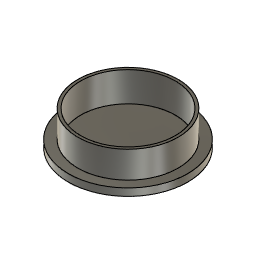
PVC End Cap v1 (Autodesk Fusion 360 design; units mm, degrees)
Autodesk Fusion 360 part; units mm, degrees
sketch "Sketch1" plane through (0, 0, 0) normal (0, 0, 1) x (1, 0, 0)
  circle A0 centre (0, 0) radius 30.235
  dimension "d1" = 60.47
  constraint coincident A0.centre origin
  measures "d1" diameter of A0
extrude "Extrude1" add sketch "Sketch1" along normal blind 3.72
sketch "Sketch2" plane through (0, 0, 3.72) normal (0, 0, 1) x (-1, 0, 0)
  circle A0 centre (0, 0) radius 30.235
  circle A1 centre (0, 0) radius 25.4
  dimension "d4" = 50.8
  constraint coincident A0.centre A1.centre
  measures "d4" diameter of A1
extrude "Extrude2" add sketch "Sketch2" along normal blind 13.57 contours A1
sketch "Sketch3" plane through (0, 0, 17.29) normal (0, 0, 1) x (-1, 0, 0)
  circle A0 centre (0, 0) radius 25.4
  circle A1 centre (0, 0) radius 24
  dimension "d10" = 48
  constraint coincident A0.centre A1.centre
  measures "d10" diameter of A1
extrude "Extrude3" cut sketch "Sketch3" against normal blind 15 contours A1
